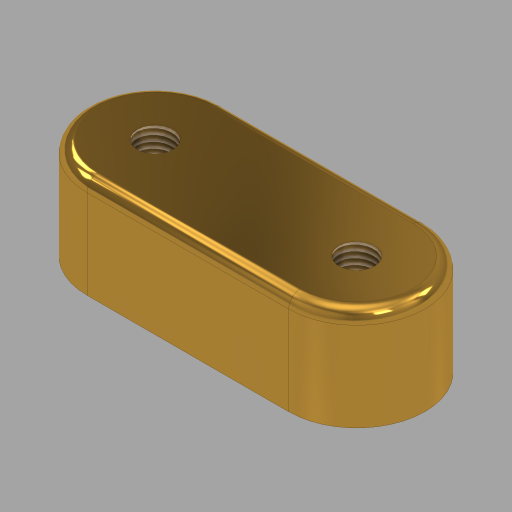
# Autodesk Inventor part: SolderSupportDoubleNut
Saved by Autodesk Inventor 2024 (Build 280153020, 153B)
## iProperties
Created: 2023-09-27
Part Number: SolderSupportDoubleNut
Material: Brass
Document SubType Name: Modeling
Designer: schanen
Density: 8.49 g/cm^3
Appearance: Brass - Polished
Author: schanen
Autodesk Inventor part; units mm, degrees
ref_plane "YZ Plane" through (0, 0, 0) normal (1, 0, 0) x (0, 1, 0)
ref_plane "XZ Plane" through (0, 0, 0) normal (0, 1, 0) x (-1, 0, 0)
ref_plane "XY Plane" through (0, 0, 0) normal (0, 0, 1) x (1, 0, 0)
sketch "Sketch1" plane through (0, 0, 0) normal (0, 1, 0) x (-1, 0, 0)
  line L0 (8.5, 0) -> (-8.5, 0) construction
  line L1 (8.5, 5.75) -> (-8.5, 5.75)
  line L2 (-8.5, -5.75) -> (8.5, -5.75)
  arc A0 (8.5, -5.75) -> (8.5, 5.75) centre (8.5, 0) ccw
  arc A1 (-8.5, 5.75) -> (-8.5, -5.75) centre (-8.5, 0) ccw
  circle A2 centre (-8.5, 0) radius 1.5
  circle A3 centre (8.5, 0) radius 1.5
  point P0 (0, 0)
  dimension "d0" = 11.5
  dimension "d1" = 17
  dimension "d2" = 3
  dimension "d3" = 3
  constraints: 8 end point, 4 centre point, 4 point on circle, 4 tangent, 2 coincident, 1 horizontal, 1 midpoint, 1 parallel
  measures "d0" diameter of A1
  measures "d1" distance of L0.start L0.end
  measures "d2" diameter of A2
  measures "d3" diameter of A3
extrude "Extrusion1" add sketch "Sketch1" along normal blind 8.5
thread "Thread1" size "M3x0.5" class "6H" standard "ANSI Metric M Profile" length 11.5
thread "Thread2" size "M3x0.5" class "6H" standard "ANSI Metric M Profile" length 11.5
fillet "Fillet1" radius 1 4 edges at (0, 8.5, 5.75) (14.25, 8.5, 0) (0, 8.5, -5.75) (-14.25, 8.5, 0)
body "Solid1"
